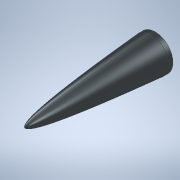
# Autodesk Inventor part: nose
Saved by Autodesk Inventor 2020 (Build 240168000, 168)
## iProperties
Created: 2021-01-23
Part Number: nose
Material: ABS Plastic
Document SubType Name: Modeling
Designer: 0x6f736f646f
Density: 1.06 g/cm^3
Appearance: Iron Gray
Author: 0x6f736f646f
Autodesk Inventor part; units mm, degrees
ref_plane "YZ Plane" through (0, 0, 0) normal (1, 0, 0) x (0, 1, 0)
ref_plane "XZ Plane" through (0, 0, 0) normal (0, 1, 0) x (-1, 0, 0)
ref_plane "XY Plane" through (0, 0, 0) normal (0, 0, 1) x (1, 0, 0)
sketch "Sketch1" plane through (0, 0, 0) normal (1, 0, 0) x (0, 1, 0)
  spline S0 degree 2 poles (16.8, 0) (7.4765, 120) (0, 120) knots 0 0 0 1 1 1
  spline S1 degree 2 poles (15, 0) (6.5777, 118.2) (0, 118.2) knots 0 0 0 1 1 1
  line L0 (0, 146.91) -> (0, -29.1517) projected
  line L1 (0, 120) -> (0, 118.2)
  line L2 (0.9491, 118.2) -> (-0.9491, 118.2) construction
  arc A0 (0.527, 117.976) -> (-0.527, 117.976) centre (0, 117.4679) ccw construction
  line L3 (1.0883, 120) -> (-1.0883, 120) construction
  arc A1 (0.6361, 119.749) -> (-0.6361, 119.749) centre (0, 119.0684) ccw construction
  line L4 (16.8, 0) -> (16.8, -4)
  line L5 (16.8, -4) -> (15, -4)
  line L6 (15, -4) -> (15, 0)
  dimension "d62" = 15
  dimension "d63" = 1.8
  dimension "d64" = 118.2
  dimension "d65" = 120
  constraints: 12 end point, 4 midpoint, 2 centre point, 2 horizontal, 2 perpendicular, 2 point on circle, 2 point on line, 1 vertical, 7 other
  measures "d62" distance from line of L0 L6.end
  measures "d63" distance of L4.end L5.end
  measures "d64" vertical distance of L1.end L6.end
  measures "d65" vertical distance of L1.start L4.start
revolve "Revolution4" add sketch "Sketch1" angle 360 about axis through (0, 0, 0) along (0, 0, -1)
body "Solid3"
